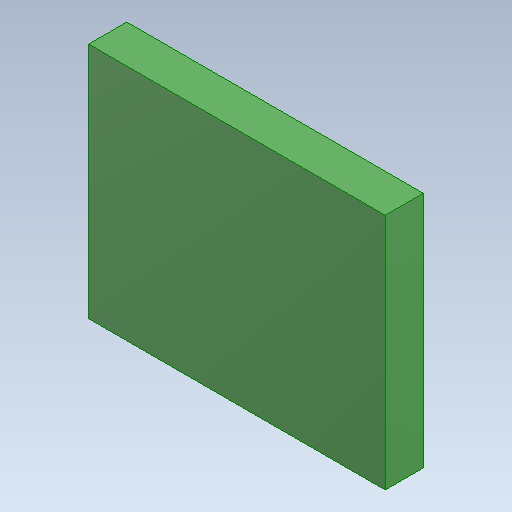
# Autodesk Inventor part: TCA9548APWR
Saved by Autodesk Inventor 2020 (Build 240168000, 168)
## iProperties
Created: 2019-05-24
Part Number: TCA9548APWR
Material: Generic
Document SubType Name: Modeling
Designer: psrob
Density: 1 g/cm^3
Appearance: TSSOP24, TCA9548APWR
Author: psrob
Autodesk Inventor part; units mm, degrees
ref_plane "YZ Plane" through (0, 0, 0) normal (1, 0, 0) x (0, 1, 0)
ref_plane "XZ Plane" through (0, 0, 0) normal (0, 1, 0) x (-1, 0, 0)
ref_plane "XY Plane" through (0, 0, 0) normal (0, 0, 1) x (1, 0, 0)
sketch "TSSOP24, TCA9548APWR_61" plane through (0, 0, 0) normal (0, 0, 1) x (1, 0, 0)
  line L0 (-3.8908, 3.121) -> (3.8908, 3.121)
  line L1 (3.8908, 3.121) -> (3.8908, -3.121)
  line L2 (3.8908, -3.121) -> (-3.8908, -3.121)
  line L3 (-3.8908, -3.121) -> (-3.8908, 3.121)
  constraints: 8 end point
extrude "Extrusion1" add sketch "TSSOP24, TCA9548APWR_61" along normal blind 1
body "Solid1"
